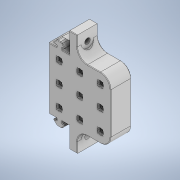
# Autodesk Inventor part: 9inSpacer
Saved by Autodesk Inventor 2020 (Build 240168000, 168)
## iProperties
Created: 2020-01-07
Part Number: 9inSpacer
Material: Generic
Document SubType Name: Modeling
Designer: srini
Density: 1 g/cm^3
Appearance: Default
Author: srini
Autodesk Inventor part; units mm, degrees
ref_plane "YZ Plane" through (0, 0, 0) normal (1, 0, 0) x (0, 1, 0)
ref_plane "XZ Plane" through (0, 0, 0) normal (0, 1, 0) x (-1, 0, 0)
ref_plane "XY Plane" through (0, 0, 0) normal (0, 0, 1) x (1, 0, 0)
sketch "Sketch1" plane through (0, 0, 0) normal (0, 0, 1) x (1, 0, 0)
  line L0 (-267.5181, -12.7) -> (-258.3363, -12.7)
  line L1 (11.8819, -12.7) -> (11.8819, -88.9)
  line L2 (11.8819, -88.9) -> (2.7, -88.9)
  line L3 (-267.5181, -88.9) -> (-267.5181, -12.7)
  line L4 (-267.5181, -6.3246) -> (-267.5181, -9.5504) construction
  line L5 (-248.4935, -12.7) -> (-245.2677, -12.7) construction
  line L6 (-261.1427, -88.9) -> (-264.3685, -88.9) construction
  line L7 (11.8819, -9.5504) -> (11.8819, -6.3246) construction
  line L8 (-13.5181, 5.3086) -> (-13.5181, -5.3086) construction
  line L9 (-7.1427, 12.7) -> (-10.3685, 12.7) construction
  line L10 (-242.1181, -5.3086) -> (-242.1181, 5.3086) construction
  arc A0 (-259.1204, -12.7) -> (-259.1204, -10.4902) centre (-259.1204, -11.5951) ccw construction
  line L11 (-259.1204, -10.4902) -> (-261.2929, -10.4902) construction
  arc A1 (-262.0113, -8.7558) -> (-261.2929, -10.4902) centre (-261.2929, -9.4742) ccw construction
  line L12 (-262.0113, -8.7558) -> (-258.694, -5.4384) construction
  arc A2 (-256.4489, -4.5085) -> (-258.694, -5.4384) centre (-256.4489, -7.6835) ccw construction
  line L13 (-256.4489, -4.5085) -> (-253.1873, -4.5085) construction
  arc A3 (-250.9423, -5.4384) -> (-253.1873, -4.5085) centre (-253.1873, -7.6835) ccw construction
  line L14 (-250.9423, -5.4384) -> (-247.6249, -8.7558) construction
  arc A4 (-248.3433, -10.4902) -> (-247.6249, -8.7558) centre (-248.3433, -9.4742) ccw construction
  line L15 (-248.3433, -10.4902) -> (-250.5158, -10.4902) construction
  arc A5 (-250.5158, -10.4902) -> (-250.5158, -12.7) centre (-250.5158, -11.5951) ccw construction
  arc A6 (-259.1204, -91.1098) -> (-259.1204, -88.9) centre (-259.1204, -90.0049) ccw construction
  line L16 (-261.2929, -91.1098) -> (-259.1204, -91.1098) construction
  arc A7 (-261.2929, -91.1098) -> (-262.0113, -92.8442) centre (-261.2929, -92.1258) ccw construction
  line L17 (-258.694, -96.1616) -> (-262.0113, -92.8442) construction
  arc A8 (-258.694, -96.1616) -> (-256.4489, -97.0915) centre (-256.4489, -93.9165) ccw construction
  line L18 (-253.1873, -97.0915) -> (-256.4489, -97.0915) construction
  arc A9 (-253.1873, -97.0915) -> (-250.9423, -96.1616) centre (-253.1873, -93.9165) ccw construction
  line L19 (-247.6249, -92.8442) -> (-250.9423, -96.1616) construction
  arc A10 (-247.6249, -92.8442) -> (-248.3433, -91.1098) centre (-248.3433, -92.1258) ccw construction
  line L20 (-250.5158, -91.1098) -> (-248.3433, -91.1098) construction
  arc A11 (-250.5158, -88.9) -> (-250.5158, -91.1098) centre (-250.5158, -90.0049) ccw construction
  arc A12 (-5.1204, -12.7) -> (-5.1204, -10.4902) centre (-5.1204, -11.5951) ccw construction
  line L21 (-5.1204, -10.4902) -> (-7.2929, -10.4902) construction
  arc A13 (-8.0113, -8.7558) -> (-7.2929, -10.4902) centre (-7.2929, -9.4742) ccw construction
  line L22 (-8.0113, -8.7558) -> (-4.694, -5.4384) construction
  arc A14 (-2.4489, -4.5085) -> (-4.694, -5.4384) centre (-2.4489, -7.6835) ccw construction
  line L23 (-2.4489, -4.5085) -> (0.8127, -4.5085) construction
  arc A15 (3.0577, -5.4384) -> (0.8127, -4.5085) centre (0.8127, -7.6835) ccw construction
  line L24 (3.0577, -5.4384) -> (6.3751, -8.7558) construction
  arc A16 (5.6567, -10.4902) -> (6.3751, -8.7558) centre (5.6567, -9.4742) ccw construction
  line L25 (5.6567, -10.4902) -> (3.4842, -10.4902) construction
  arc A17 (3.4842, -10.4902) -> (3.4842, -12.7) centre (3.4842, -11.5951) ccw construction
  arc A18 (-5.1204, -91.1098) -> (-5.1204, -88.9) centre (-5.1204, -90.0049) ccw construction
  line L26 (-7.2929, -91.1098) -> (-5.1204, -91.1098) construction
  arc A19 (-7.2929, -91.1098) -> (-8.0113, -92.8442) centre (-7.2929, -92.1258) ccw construction
  line L27 (-4.694, -96.1616) -> (-8.0113, -92.8442) construction
  arc A20 (-4.694, -96.1616) -> (-2.4489, -97.0915) centre (-2.4489, -93.9165) ccw construction
  line L28 (0.8127, -97.0915) -> (-2.4489, -97.0915) construction
  arc A21 (0.8127, -97.0915) -> (3.0577, -96.1616) centre (0.8127, -93.9165) ccw construction
  line L29 (6.3751, -92.8442) -> (3.0577, -96.1616) construction
  arc A22 (6.3751, -92.8442) -> (5.6567, -91.1098) centre (5.6567, -92.1258) ccw construction
  line L30 (3.4842, -91.1098) -> (5.6567, -91.1098) construction
  arc A23 (3.4842, -88.9) -> (3.4842, -91.1098) centre (3.4842, -90.0049) ccw construction
  arc A24 (-4.3363, -12.7) -> (-5.1204, -10.2402) centre (-5.1204, -11.5951) ccw
  line L31 (-5.1204, -10.2402) -> (-7.2929, -10.2402)
  arc A25 (-7.8346, -8.9326) -> (-7.2929, -10.2402) centre (-7.2929, -9.4742) ccw
  line L32 (-7.8346, -8.9326) -> (-4.5172, -5.6152)
  arc A26 (-2.4489, -4.7585) -> (-4.5172, -5.6152) centre (-2.4489, -7.6835) ccw
  line L33 (-2.4489, -4.7585) -> (0.8127, -4.7585)
  arc A27 (2.881, -5.6152) -> (0.8127, -4.7585) centre (0.8127, -7.6835) ccw
  line L34 (2.881, -5.6152) -> (6.1983, -8.9326)
  arc A28 (5.6567, -10.2402) -> (6.1983, -8.9326) centre (5.6567, -9.4742) ccw
  line L35 (5.6567, -10.2402) -> (3.4842, -10.2402)
  arc A29 (3.4842, -10.2402) -> (2.7, -12.7) centre (3.4842, -11.5951) ccw
  arc A30 (-5.1204, -91.3598) -> (-4.3363, -88.9) centre (-5.1204, -90.0049) ccw
  line L36 (-5.1204, -91.3598) -> (-7.2929, -91.3598)
  arc A31 (-7.2929, -91.3598) -> (-7.8346, -92.6674) centre (-7.2929, -92.1258) ccw
  line L37 (-7.8346, -92.6674) -> (-4.5172, -95.9848)
  arc A32 (-4.5172, -95.9848) -> (-2.4489, -96.8415) centre (-2.4489, -93.9165) ccw
  line L38 (-2.4489, -96.8415) -> (0.8127, -96.8415)
  arc A33 (0.8127, -96.8415) -> (2.881, -95.9848) centre (0.8127, -93.9165) ccw
  line L39 (2.881, -95.9848) -> (6.1983, -92.6674)
  arc A34 (6.1983, -92.6674) -> (5.6567, -91.3598) centre (5.6567, -92.1258) ccw
  line L40 (5.6567, -91.3598) -> (3.4842, -91.3598)
  arc A35 (2.7, -88.9) -> (3.4842, -91.3598) centre (3.4842, -90.0049) ccw
  arc A36 (-259.1204, -91.3598) -> (-258.3363, -88.9) centre (-259.1204, -90.0049) ccw
  line L41 (-259.1204, -91.3598) -> (-261.2929, -91.3598)
  arc A37 (-261.2929, -91.3598) -> (-261.8346, -92.6674) centre (-261.2929, -92.1258) ccw
  line L42 (-261.8346, -92.6674) -> (-258.5172, -95.9848)
  arc A38 (-258.5172, -95.9848) -> (-256.4489, -96.8415) centre (-256.4489, -93.9165) ccw
  line L43 (-256.4489, -96.8415) -> (-253.1873, -96.8415)
  arc A39 (-253.1873, -96.8415) -> (-251.119, -95.9848) centre (-253.1873, -93.9165) ccw
  line L44 (-251.119, -95.9848) -> (-247.8017, -92.6674)
  arc A40 (-247.8017, -92.6674) -> (-248.3433, -91.3598) centre (-248.3433, -92.1258) ccw
  line L45 (-248.3433, -91.3598) -> (-250.5158, -91.3598)
  arc A41 (-251.3, -88.9) -> (-250.5158, -91.3598) centre (-250.5158, -90.0049) ccw
  arc A42 (-258.3363, -12.7) -> (-259.1204, -10.2402) centre (-259.1204, -11.5951) ccw
  line L46 (-259.1204, -10.2402) -> (-261.2929, -10.2402)
  arc A43 (-261.8346, -8.9326) -> (-261.2929, -10.2402) centre (-261.2929, -9.4742) ccw
  line L47 (-261.8346, -8.9326) -> (-258.5172, -5.6152)
  arc A44 (-256.4489, -4.7585) -> (-258.5172, -5.6152) centre (-256.4489, -7.6835) ccw
  line L48 (-256.4489, -4.7585) -> (-253.1873, -4.7585)
  arc A45 (-251.119, -5.6152) -> (-253.1873, -4.7585) centre (-253.1873, -7.6835) ccw
  line L49 (-251.119, -5.6152) -> (-247.8017, -8.9326)
  arc A46 (-248.3433, -10.2402) -> (-247.8017, -8.9326) centre (-248.3433, -9.4742) ccw
  line L50 (-248.3433, -10.2402) -> (-250.5158, -10.2402)
  arc A47 (-250.5158, -10.2402) -> (-251.3, -12.7) centre (-250.5158, -11.5951) ccw
  line L51 (-258.3363, -88.9) -> (-267.5181, -88.9)
  line L52 (-251.3, -88.9) -> (-258.3363, -88.9)
  line L53 (-258.3363, -12.7) -> (-251.3, -12.7)
  line L54 (-251.3, -12.7) -> (-4.3363, -12.7)
  line L55 (-4.3363, -12.7) -> (2.7, -12.7)
  line L56 (2.7, -12.7) -> (11.8819, -12.7)
  line L57 (-4.3363, -88.9) -> (-251.3, -88.9)
  line L58 (2.7, -88.9) -> (-4.3363, -88.9)
  line L59 (-49.7931, -12.7) -> (-13.5181, 12.7)
  line L60 (-13.5181, 12.7) -> (-13.5181, -12.7)
  line L61 (-13.5181, -12.7) -> (-49.7931, -12.7)
  line L62 (-49.7931, -88.9) -> (-13.5181, -114.3)
  line L63 (-13.5181, -114.3) -> (-13.5181, -88.9)
  line L64 (-13.5181, -88.9) -> (-49.7931, -88.9)
  line L65 (-242.1181, 12.7) -> (-242.1181, -12.7)
  line L66 (-242.1181, -12.7) -> (-205.8432, -12.7)
  line L67 (-205.8432, -12.7) -> (-242.1181, 12.7)
  line L68 (-242.1181, -88.9) -> (-242.1181, -114.3)
  line L69 (-242.1181, -114.3) -> (-205.8432, -88.9)
  line L70 (-205.8432, -88.9) -> (-242.1181, -88.9)
  line L71 (-261.1427, 12.7) -> (-264.3685, 12.7) projected
  line L72 (-242.1181, -114.3) -> (-232.5931, -114.3)
  line L73 (-232.5931, -114.3) -> (-232.5931, -88.9)
  line L74 (-232.5931, -88.9) -> (-242.1181, -88.9)
  line L75 (-242.1181, -88.9) -> (-242.1181, -114.3)
  line L76 (-242.1181, -12.7) -> (-232.5931, -12.7)
  line L77 (-232.5931, -12.7) -> (-232.5931, 12.7)
  line L78 (-232.5931, 12.7) -> (-242.1181, 12.7)
  line L79 (-242.1181, 12.7) -> (-242.1181, -12.7)
  point P0 (0, 0)
  point P1 (-13.5181, -12.7)
  point P2 (-49.7931, -12.7)
  point P3 (-205.8432, -88.9)
  point P4 (-49.7931, -88.9)
  point P5 (-232.5931, 6.0305)
  point P6 (-232.5931, -107.6305)
  point P7 (-232.5931, -12.7)
  point P8 (-232.5931, -88.9)
  dimension "d0" = 0.25
  dimension "d1" = 0.25
  dimension "d2" = 0.25
  dimension "d3" = 0.25
  dimension "d4" = 145
  dimension "d22" = 9.525
  constraints: 104 end point, 48 point on circle, 31 parallel, 24 centre point, 14 collinear, 14 tangent, 9 perpendicular, 7 horizontal, 6 equal length, 6 point on line, 1 vertical, 36 other
  measures "d0" distance between parallel lines of L48 L13
  measures "d1" distance between parallel lines of L33 L23
  measures "d2" distance between parallel lines of L38 L28
  measures "d3" distance between parallel lines of L43 L18
  measures "d4" angle of L67 L54
  measures "d22" distance of L72.start L72.end
extrude "Extrusion1" add sketch "Sketch1" against normal blind 25.4 contours L0 L53 L54 L55 L56 L1 L2 L58 L57 L52 L51 L3 | A42 L46 A43 L47 A44 L48 A45 L49 A46 L50 A47 L53 | L52 A41 L45 A40 L44 A39 L43 A38 L42 A37 L41 A36 | L65 L67 L77 L54 | L78 L77 L67 | L57 L73 L69 L68 | L69 L73 L72 | L59 L60 L54 | L57 L63 L62 | A24 L31 A25 L32 A26 L33 A27 L34 A28 L35 A29 L55 | L58 A35 L40 A34 L39 A33 L38 A32 L37 A31 L36 A30
sketch "Sketch3" plane through (0, 0, 0) normal (0, 0, 1) x (1, 0, 0)
  circle A0 centre (-254.8181, -76.2) radius 3.3734
  circle A1 centre (-254.8181, -101.6) radius 2.6035 projected
  line L0 (-267.5181, -12.7) -> (-267.5181, -88.9) projected
  line L1 (-267.5181, -88.9) -> (-258.3363, -88.9) projected
  circle A2 centre (-254.8181, -50.8) radius 3.3734
  circle A3 centre (-254.8181, -25.4) radius 3.3734
  circle A4 centre (-229.4181, -76.2) radius 3.3734
  circle A5 centre (-229.4181, -50.8) radius 3.3734
  circle A6 centre (-229.4181, -25.4) radius 3.3734
  circle A7 centre (-204.0181, -76.2) radius 3.3734
  circle A8 centre (-204.0181, -50.8) radius 3.3734
  circle A9 centre (-204.0181, -25.4) radius 3.3734
  point P0 (0, 0)
  dimension "d7" = 6.7469
  dimension "d8" = 25.4
  dimension "d11" = 25.4
  dimension "d14" = 25.4
  constraints: 9 centre point, 1 horizontal, 1 vertical, 1 vertical alignment, 16 other
  measures "d7" diameter of A0
  measures "d8" distance of A0.centre A1.centre
  measures "d11" distance of A0.centre A2.centre
  measures "d14" distance of A0.centre A4.centre
extrude "Extrusion2" cut sketch "Sketch3" against normal through all contours A0 | A2 | A3 | A4 | A5 | A6 | A7 | A8 | A9
sketch "Sketch4" plane through (0, 0, 0) normal (0, 0, 1) x (1, 0, 0)
  line L0 (-191.3181, -132.299) -> (29.4064, -132.299)
  line L1 (29.4064, -132.299) -> (29.4064, 59.0917)
  line L2 (29.4064, 59.0917) -> (-191.3181, 59.0917)
  line L3 (-191.3181, 59.0917) -> (-191.3181, -132.299)
  line L4 (-242.1181, -88.9) -> (-242.1181, -114.3) projected
  point P0 (0, 0)
  dimension "d19" = 50.8
  constraints: 8 end point, 2 parallel, 1 horizontal, 1 perpendicular
  measures "d19" distance between parallel lines of L3 L4
extrude "Extrusion3" cut sketch "Sketch4" against normal through all
sketch "Sketch5" plane through (-242.1181, -114.3, 0) normal (-1, 0, 0) x (0, 0, 1)
  circle A0 centre (-12.7, 12.7) radius 3.3734
  line L0 (0, 0) -> (-25.4, 0) projected
  line L1 (-25.4, 0) -> (-25.4, 25.4) projected
  circle A1 centre (-12.7, 114.3) radius 3.3734
  point P0 (0, 114.3)
  dimension "d23" = 12.7
  dimension "d24" = 12.7
  dimension "d25" = 6.7469
  dimension "d28" = 101.6
  constraints: 2 centre point, 1 vertical, 2 other
  measures "d23" distance from line of A0.centre L0
  measures "d24" distance from line of A0.centre L1
  measures "d25" diameter of A0
  measures "d28" distance of A0.centre A1.centre
extrude "Extrusion4" cut sketch "Sketch5" against normal blind 25.4
fillet "Fillet1" radius 12.7 2 edges at (-232.5931, -88.9, -12.7) (-232.5931, -12.7, -12.7)
fillet "Fillet2" radius 12.7 2 edges at (-191.3181, -88.9, -12.7) (-191.3181, -12.7, -12.7)
chamfer "Chamfer1" distance 0.635 angle 45 98 edges at (-232.5931, -107.95, 0) (-228.8734, -92.6197, 0) (-211.9556, -88.9, 0) (-195.0379, -85.1803, 0) (-191.3181, -50.8, 0) (-195.0379, -16.4197, 0) (-211.9556, -12.7, 0) (-228.8734, -8.9803, 0) (-232.5931, 6.35, 0) (-237.3556, -114.3, 0) (-242.1181, -101.6, 0) (-246.7091, -88.9, 0) (-251.8067, -90.4164, 0) (-249.4296, -91.3598, 0) (-247.6356, -91.8327, 0) (-249.4604, -94.3261, 0) (-252.068, -96.6188, 0) (-254.8181, -96.8415, 0) (-257.5683, -96.6188, 0) (-260.1759, -94.3261, 0) (-262.0006, -91.8327, 0) (-260.2067, -91.3598, 0) (-257.8296, -90.4164, 0) (-262.9272, -88.9, 0) (-267.5181, -50.8, 0) (-237.3556, 12.7, 0) (-242.1181, 0, 0) (-246.7091, -12.7, 0) (-251.8067, -11.1836, 0) (-249.4296, -10.2402, 0) (-247.6356, -9.7673, 0) (-249.4604, -7.2739, 0) (-252.068, -4.9812, 0) (-254.8181, -4.7585, 0) (-257.5683, -4.9812, 0) (-260.1759, -7.2739, 0) (-262.0006, -9.7673, 0) (-260.2067, -10.2402, 0) (-257.8296, -11.1836, 0) (-262.9272, -12.7, 0) (-258.1916, -25.4, 0) (-232.7916, -25.4, 0) (-207.3916, -25.4, 0) (-207.3916, -50.8, 0) (-232.7916, -50.8, 0) (-258.1916, -50.8, 0) (-258.1916, -76.2, 0) (-232.7916, -76.2, 0) (-207.3916, -76.2, 0) (-207.3916, -76.2, -25.4) (-207.3916, -50.8, -25.4) (-207.3916, -25.4, -25.4) (-232.7916, -25.4, -25.4) (-232.7916, -50.8, -25.4) (-232.7916, -76.2, -25.4) (-258.1916, -76.2, -25.4) (-258.1916, -50.8, -25.4) (-258.1916, -25.4, -25.4) (-249.4296, -10.2402, -25.4) (-251.8067, -11.1836, -25.4) (-247.6356, -9.7673, -25.4) (-249.4604, -7.2739, -25.4) (-252.068, -4.9812, -25.4) (-254.8181, -4.7585, -25.4) (-257.5683, -4.9812, -25.4) (-260.1759, -7.2739, -25.4) (-262.0006, -9.7673, -25.4) (-260.2067, -10.2402, -25.4) (-257.8296, -11.1836, -25.4) (-246.7091, -12.7, -25.4) (-262.9272, -12.7, -25.4) (-246.7091, -88.9, -25.4) (-249.4296, -91.3598, -25.4) (-247.6356, -91.8327, -25.4) (-249.4604, -94.3261, -25.4) (-252.068, -96.6188, -25.4) (-254.8181, -96.8415, -25.4) (-257.5683, -96.6188, -25.4) (-260.1759, -94.3261, -25.4) (-262.0006, -91.8327, -25.4) (-260.2067, -91.3598, -25.4) (-257.8296, -90.4164, -25.4) (-251.8067, -90.4164, -25.4) (-262.9272, -88.9, -25.4) (-267.5181, -50.8, -25.4) (-242.1181, 0, -25.4) (-237.3556, 12.7, -25.4) (-232.5931, 6.35, -25.4) (-228.8734, -8.9803, -25.4) (-211.9556, -12.7, -25.4) (-195.0379, -16.4197, -25.4) (-191.3181, -50.8, -25.4) (-195.0379, -85.1803, -25.4) (-211.9556, -88.9, -25.4) (-228.8734, -92.6197, -25.4) (-232.5931, -107.95, -25.4) (-237.3556, -114.3, -25.4) (-242.1181, -101.6, -25.4)
sketch "Sketch8" plane through (-242.1181, -114.3, -24.765) normal (-1, 0, 0) x (0, 0, 1)
  line L0 (15.4384, 16.0734) -> (8.6916, 16.0734)
  line L1 (8.6916, 16.0734) -> (8.6916, 9.3266)
  line L2 (8.6916, 9.3266) -> (15.4384, 9.3266)
  line L3 (15.4384, 9.3266) -> (15.4384, 16.0734)
  circle A0 centre (12.065, 12.7) radius 3.3734 projected
  line L4 (15.4384, 16.0734) -> (8.6916, 9.3266) construction
  line L5 (8.6916, 16.0734) -> (15.4384, 9.3266) construction
  line L6 (15.4384, 117.6734) -> (8.6916, 117.6734)
  line L7 (8.6916, 117.6734) -> (8.6916, 110.9266)
  line L8 (8.6916, 110.9266) -> (15.4384, 110.9266)
  line L9 (15.4384, 110.9266) -> (15.4384, 117.6734)
  arc A1 (15.4384, 114.3) -> (8.6916, 114.3) centre (12.065, 114.3) ccw projected
  line L10 (15.4384, 117.6734) -> (8.6916, 110.9266) construction
  line L11 (8.6916, 117.6734) -> (15.4384, 110.9266) construction
  point P0 (24.765, 114.3)
  constraints: 24 end point, 4 midpoint, 4 parallel, 4 tangent, 2 horizontal, 2 perpendicular
extrude "Extrusion6" cut sketch "Sketch8" against normal blind 3.175
sketch "Sketch9" plane through (-242.1181, -114.3, -24.765) normal (-1, 0, 0) x (0, 0, 1)
  arc A0 (8.6916, 12.7) -> (15.4384, 12.7) centre (12.065, 12.7) ccw projected
  circle A1 centre (12.065, 12.7) radius 7.62
  arc A2 (15.4384, 114.3) -> (8.6916, 114.3) centre (12.065, 114.3) ccw projected
  circle A3 centre (12.065, 114.3) radius 7.62
  point P0 (24.765, 114.3)
  dimension "d45" = 15.24
  constraints: 2 centre point, 2 coincident, 1 equal radius
  measures "d45" diameter of A3
extrude "Extrusion7" cut sketch "Sketch9" along normal through all
sketch "Sketch10" plane through (-232.5931, -101.6, -12.7) normal (1, 0, 0) x (0, 0, -1)
  arc A0 (-3.3734, 0) -> (3.3734, 0) centre (0, 0) ccw projected
  circle A1 centre (0, 0) radius 7.62
  arc A2 (3.3734, 101.6) -> (-3.3734, 101.6) centre (0, 101.6) ccw projected
  circle A3 centre (0, 101.6) radius 7.62
  point P0 (-12.7, 101.6)
  dimension "d48" = 15.24
  constraints: 2 centre point, 2 coincident, 1 equal radius
  measures "d48" diameter of A1
extrude "Extrusion8" cut sketch "Sketch10" along normal through all
fillet "Fillet3" radius 0.9525 2 edges at (-242.1181, -88.9, -12.7) (-242.1181, -12.7, -12.7)
sketch "Sketch11" plane through (0, 0, 0) normal (0, 0, 1) x (1, 0, 0)
  line L0 (-251.4447, -72.8266) -> (-258.1916, -72.8266)
  line L1 (-258.1916, -72.8266) -> (-258.1916, -79.5734)
  line L2 (-258.1916, -79.5734) -> (-251.4447, -79.5734)
  line L3 (-251.4447, -79.5734) -> (-251.4447, -72.8266)
  circle A0 centre (-254.8181, -76.2) radius 3.3734 projected
  line L4 (-251.4447, -72.8266) -> (-258.1916, -79.5734) construction
  line L5 (-258.1916, -72.8266) -> (-251.4447, -79.5734) construction
  line L6 (-232.7916, -79.5734) -> (-226.0447, -79.5734)
  line L7 (-232.7916, -72.8266) -> (-232.7916, -79.5734)
  line L8 (-226.0447, -79.5734) -> (-226.0447, -72.8266)
  line L9 (-226.0447, -72.8266) -> (-232.7916, -72.8266)
  line L10 (-207.3916, -79.5734) -> (-200.6447, -79.5734)
  line L11 (-207.3916, -72.8266) -> (-207.3916, -79.5734)
  line L12 (-200.6447, -79.5734) -> (-200.6447, -72.8266)
  line L13 (-200.6447, -72.8266) -> (-207.3916, -72.8266)
  line L14 (-258.1916, -54.1734) -> (-251.4447, -54.1734)
  line L15 (-258.1916, -47.4266) -> (-258.1916, -54.1734)
  line L16 (-251.4447, -54.1734) -> (-251.4447, -47.4266)
  line L17 (-251.4447, -47.4266) -> (-258.1916, -47.4266)
  line L18 (-232.7916, -54.1734) -> (-226.0447, -54.1734)
  line L19 (-232.7916, -47.4266) -> (-232.7916, -54.1734)
  line L20 (-226.0447, -54.1734) -> (-226.0447, -47.4266)
  line L21 (-226.0447, -47.4266) -> (-232.7916, -47.4266)
  line L22 (-207.3916, -54.1734) -> (-200.6447, -54.1734)
  line L23 (-207.3916, -47.4266) -> (-207.3916, -54.1734)
  line L24 (-200.6447, -54.1734) -> (-200.6447, -47.4266)
  line L25 (-200.6447, -47.4266) -> (-207.3916, -47.4266)
  line L26 (-258.1916, -28.7734) -> (-251.4447, -28.7734)
  line L27 (-258.1916, -22.0266) -> (-258.1916, -28.7734)
  line L28 (-251.4447, -28.7734) -> (-251.4447, -22.0266)
  line L29 (-251.4447, -22.0266) -> (-258.1916, -22.0266)
  line L30 (-232.7916, -28.7734) -> (-226.0447, -28.7734)
  line L31 (-232.7916, -22.0266) -> (-232.7916, -28.7734)
  line L32 (-226.0447, -28.7734) -> (-226.0447, -22.0266)
  line L33 (-226.0447, -22.0266) -> (-232.7916, -22.0266)
  line L34 (-207.3916, -28.7734) -> (-200.6447, -28.7734)
  line L35 (-207.3916, -22.0266) -> (-207.3916, -28.7734)
  line L36 (-200.6447, -28.7734) -> (-200.6447, -22.0266)
  line L37 (-200.6447, -22.0266) -> (-207.3916, -22.0266)
  point P0 (0, 0)
  dimension "d54" = 25.4
  dimension "d57" = 25.4
  constraints: 76 end point, 2 collinear, 2 horizontal, 2 midpoint, 2 parallel, 2 tangent, 1 perpendicular, 1 vertical, 62 other
  measures "d54" distance of L1.end L6.start
  measures "d57" distance of L1.end L14.start
extrude "Extrusion9" cut sketch "Sketch11" against normal blind 3.175
sketch "Sketch12" plane through (0, 0, -25.4) normal (0, 0, -1) x (-1, 0, 0)
  line L0 (251.4447, -22.0266) -> (258.1916, -22.0266)
  line L1 (258.1916, -22.0266) -> (258.1916, -28.7734)
  line L2 (258.1916, -28.7734) -> (251.4447, -28.7734)
  line L3 (251.4447, -28.7734) -> (251.4447, -22.0266)
  arc A0 (256.9832, -22.0266) -> (252.6531, -22.0266) centre (254.8181, -25.4) ccw projected
  line L4 (251.4447, -22.0266) -> (258.1916, -28.7734) construction
  line L5 (258.1916, -22.0266) -> (251.4447, -28.7734) construction
  circle A1 centre (254.8181, -25.4) radius 3.3734 projected
  line L6 (226.0447, -22.0266) -> (232.7916, -22.0266)
  line L7 (232.7916, -22.0266) -> (232.7916, -28.7734)
  line L8 (226.0447, -28.7734) -> (226.0447, -22.0266)
  line L9 (232.7916, -28.7734) -> (226.0447, -28.7734)
  line L10 (200.6447, -22.0266) -> (207.3916, -22.0266)
  line L11 (207.3916, -22.0266) -> (207.3916, -28.7734)
  line L12 (200.6447, -28.7734) -> (200.6447, -22.0266)
  line L13 (207.3916, -28.7734) -> (200.6447, -28.7734)
  line L14 (251.4447, -47.4266) -> (258.1916, -47.4266)
  line L15 (258.1916, -47.4266) -> (258.1916, -54.1734)
  line L16 (251.4447, -54.1734) -> (251.4447, -47.4266)
  line L17 (258.1916, -54.1734) -> (251.4447, -54.1734)
  line L18 (226.0447, -47.4266) -> (232.7916, -47.4266)
  line L19 (232.7916, -47.4266) -> (232.7916, -54.1734)
  line L20 (226.0447, -54.1734) -> (226.0447, -47.4266)
  line L21 (232.7916, -54.1734) -> (226.0447, -54.1734)
  line L22 (200.6447, -47.4266) -> (207.3916, -47.4266)
  line L23 (207.3916, -47.4266) -> (207.3916, -54.1734)
  line L24 (200.6447, -54.1734) -> (200.6447, -47.4266)
  line L25 (207.3916, -54.1734) -> (200.6447, -54.1734)
  line L26 (251.4447, -72.8266) -> (258.1916, -72.8266)
  line L27 (258.1916, -72.8266) -> (258.1916, -79.5734)
  line L28 (251.4447, -79.5734) -> (251.4447, -72.8266)
  line L29 (258.1916, -79.5734) -> (251.4447, -79.5734)
  line L30 (226.0447, -72.8266) -> (232.7916, -72.8266)
  line L31 (232.7916, -72.8266) -> (232.7916, -79.5734)
  line L32 (226.0447, -79.5734) -> (226.0447, -72.8266)
  line L33 (232.7916, -79.5734) -> (226.0447, -79.5734)
  line L34 (200.6447, -72.8266) -> (207.3916, -72.8266)
  line L35 (207.3916, -72.8266) -> (207.3916, -79.5734)
  line L36 (200.6447, -79.5734) -> (200.6447, -72.8266)
  line L37 (207.3916, -79.5734) -> (200.6447, -79.5734)
  point P0 (0, 0)
  point P1 (256.9832, -22.0266)
  point P2 (252.6531, -22.0266)
  dimension "d64" = 25.4
  dimension "d67" = 25.4
  constraints: 76 end point, 2 collinear, 2 horizontal, 2 midpoint, 2 parallel, 2 tangent, 1 perpendicular, 1 vertical, 62 other
  measures "d64" distance of L0.start L6.start
  measures "d67" distance of L0.start L14.start
extrude "Extrusion10" cut sketch "Sketch12" against normal blind 3.175 contours L0 A1 L3 | A1 L2 L3 | A1 | L0 L1 A1 | A1 L1 L2 | L6 L7 L9 L8 | L10 L11 L13 L12 | L14 L15 L17 L16 | L18 L19 L21 L20 | L22 L23 L25 L24 | L26 L27 L29 L28 | L30 L31 L33 L32 | L34 L35 L37 L36
equation "\"d1\" = d0"
equation "\"d2\" = d0"
equation "\"d3\" = d0"
body "Solid1"
